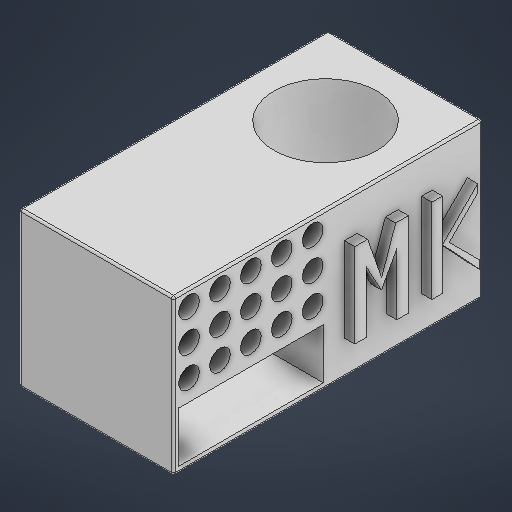
# Autodesk Inventor part: DeskOrganizer
Saved by Autodesk Inventor 2026.1 (Build 301233020, 233B)
## iProperties
Created: 2026-06-11
Part Number: DeskOrganizer
Material: Generic
Document SubType Name: Modeling
Designer: astro
Density: 1 g/cm^3
Appearance: Default
Author: astro
Autodesk Inventor part; units mm, degrees
ref_plane "YZ Plane" through (0, 0, 0) normal (1, 0, 0) x (0, 1, 0)
ref_plane "XZ Plane" through (0, 0, 0) normal (0, 1, 0) x (-1, 0, 0)
ref_plane "XY Plane" through (0, 0, 0) normal (0, 0, 1) x (1, 0, 0)
sketch "Sketch1" plane through (0, 0, 0) normal (0, 1, 0) x (-1, 0, 0)
  line L0 (0, 0) -> (150, 0)
  line L1 (150, 0) -> (150, -300)
  line L2 (150, -300) -> (0, -300)
  line L3 (0, -300) -> (0, 0)
  dimension "d0" = 150
  dimension "d1" = 300
  constraints: 8 end point, 2 parallel, 1 horizontal, 1 perpendicular
  measures "d0" distance of L1.end L2.end
  measures "d1" distance of L0.end L1.end
extrude "Extrusion1" add sketch "Sketch1" along normal blind 150
sketch "Sketch2" plane through (0, 0, 0) normal (1, 0, 0) x (0, 0, -1)
  line L0 (300, 150) -> (0, 150) projected
  line L1 (300, 0) -> (0, 0) projected
  line L2 (0, 0) -> (0, 150) projected
  circle A0 centre (15, 135) radius 10
  circle A1 centre (45, 135) radius 10
  circle A2 centre (75, 135) radius 10
  circle A3 centre (105, 135) radius 10
  circle A4 centre (135, 135) radius 10
  circle A5 centre (15, 105) radius 10
  circle A6 centre (45, 105) radius 10
  circle A7 centre (75, 105) radius 10
  circle A8 centre (105, 105) radius 10
  circle A9 centre (135, 105) radius 10
  circle A10 centre (15, 75) radius 10
  circle A11 centre (45, 75) radius 10
  circle A12 centre (75, 75) radius 10
  circle A13 centre (105, 75) radius 10
  circle A14 centre (135, 75) radius 10
  dimension "d6" = 20
  dimension "d7" = 15
  dimension "d8" = 15
  dimension "d11" = 30
  dimension "d14" = 30
  constraints: 15 centre point, 1 horizontal, 1 vertical, 28 other
  measures "d6" diameter of A0
  measures "d7" distance from line of A0.centre L2
  measures "d8" distance from line of L0 A0.centre
  measures "d11" distance of A0.centre A1.centre
  measures "d14" distance of A0.centre A5.centre
extrude "Extrusion2" cut sketch "Sketch2" against normal blind 149
sketch "Sketch3" plane through (0, 150, 0) normal (0, 1, 0) x (1, 0, 0)
  line L0 (0, 145) -> (0, 125) projected
  line L1 (0, 145) -> (-150, 145)
  line L2 (-150, 300) -> (-150, 0) projected
  circle A0 centre (-75, 222.5) radius 50
  line L3 (0, 0) -> (0, 300) projected
  line L4 (0, 300) -> (-150, 300) projected
  point P0 (-75, 145)
  point P1 (-75, 300)
  dimension "d19" = 100
  dimension "d20" = 77.5
  dimension "d21" = 75
  dimension "d22" = 77.5
  constraints: 2 end point, 2 midpoint, 1 centre point, 1 horizontal, 1 point on line
  measures "d19" diameter of A0
  measures "d20" distance of point (-75, 145) A0.centre
  measures "d21" distance from line of L3 A0.centre
  measures "d22" distance of point (-75, 300) A0.centre
extrude "Extrusion3" cut sketch "Sketch3" against normal blind 150 contours A0
sketch "Sketch4" plane through (0, 0, 0) normal (1, 0, 0) x (0, 0, -1)
  line L0 (0, 150) -> (300, 150) projected
  line L1 (150, 150) -> (150, 0)
  line L2 (300, 0) -> (0, 0) projected
  line L3 (5, 54.6089) -> (145.3394, 54.6089)
  line L4 (145.3394, 54.6089) -> (145.3394, 5.6884)
  line L5 (145.3394, 5.6884) -> (5, 5.6884)
  line L6 (5, 5.6884) -> (5, 54.6089)
  constraints: 10 end point, 2 midpoint, 2 parallel, 1 horizontal, 1 perpendicular
extrude "Extrusion4" cut sketch "Sketch4" against normal blind 149
sketch "Sketch5" plane through (0, 0, 0) normal (1, 0, 0) x (0, 0, -1)
  line L0 (165.8816, 32.9929) -> (165.8816, 114.9063)
  line L1 (165.8816, 114.9063) -> (178.3323, 114.9063)
  line L2 (178.3323, 114.9063) -> (191.9845, 75.9405)
  line L3 (191.9845, 75.9405) -> (205.6367, 114.9063)
  line L4 (205.6367, 114.9063) -> (218.0874, 114.9063)
  line L5 (218.0874, 114.9063) -> (218.0874, 32.9929)
  line L6 (218.0874, 32.9929) -> (206.6836, 32.9929)
  line L7 (206.6836, 32.9929) -> (206.6836, 92.6171)
  line L8 (206.6836, 92.6171) -> (191.8104, 65.4816)
  line L9 (191.8104, 65.4816) -> (176.9372, 92.6171)
  line L10 (176.9372, 92.6171) -> (176.9372, 32.9929)
  line L11 (165.5333, 32.9929) -> (176.9372, 32.9929)
  line L12 (218.0874, 114.9063) -> (292.5647, 114.9063)
  line L13 (240.7658, 114.9063) -> (240.7658, 32.9929)
  line L14 (240.7658, 32.9929) -> (251.0846, 32.9929)
  line L15 (251.0846, 32.9929) -> (251.0846, 114.9063)
  line L16 (240.7658, 114.9063) -> (251.0846, 114.9063)
  line L17 (251.0846, 73.9496) -> (285.275, 108.14)
  line L18 (251.0846, 73.9496) -> (299.4371, 73.9496) construction
  line L19 (285.275, 108.14) -> (285.275, 100.3411)
  line L20 (285.275, 100.3411) -> (257.5862, 72.6522)
  line L21 (257.5862, 72.6522) -> (287.5076, 42.7307)
  line L22 (287.5076, 42.7307) -> (287.5076, 34.9318)
  line L23 (287.5076, 34.9318) -> (251.0846, 73.9496)
  point P0 (0, 0)
  dimension "d27" = 45
  dimension "d28" = 90
  constraints: 48 end point, 8 equal length, 7 perpendicular, 7 point on line, 3 vertical, 2 horizontal, 2 parallel, 1 collinear, 1 midpoint
  measures "d27" angle of L18 L17
  measures "d28" angle of L21 L20
extrude "Extrusion5" add sketch "Sketch5" along normal blind 10
fillet "Fillet1" radius 2 12 edges at (0, 150, -150) (-75, 150, 0) (-150, 150, -150) (-75, 150, -300) (0, 75, 0) (-75, 0, 0) (-150, 75, 0) (0, 0, -150) (-150, 0, -150) (-75, 0, -300) (0, 75, -300) (-150, 75, -300)
shell "Shell1" thickness 1 removed faces 1 at (-75, 0, -58.8333)
body "Solid1"
